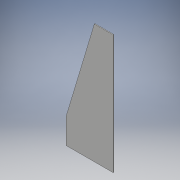
# Autodesk Inventor part: Part2
Saved by Autodesk Inventor 2018 (Build 220112000, 112)
## iProperties
Created: 2018-06-07
Part Number: Part2
Material: 一般
Document SubType Name: Modeling
Designer: ku_sk
Density: 1 g/cm^3
Appearance: 既定
Author: ku_sk
Autodesk Inventor part; units mm, degrees
ref_plane "YZ Plane" through (0, 0, 0) normal (1, 0, 0) x (0, 1, 0)
ref_plane "XZ Plane" through (0, 0, 0) normal (0, 1, 0) x (-1, 0, 0)
ref_plane "XY Plane" through (0, 0, 0) normal (0, 0, 1) x (1, 0, 0)
sketch "スケッチ1" plane through (0, 0, 0) normal (0, 1, 0) x (-1, 0, 0)
  line L0 (0, 254.5) -> (0, -254.5)
  line L1 (0, -254.5) -> (200, -254.5)
  line L2 (200, -254.5) -> (200, -145.5)
  line L3 (200, -145.5) -> (80, 254.5)
  line L4 (80, 254.5) -> (0, 254.5)
  point P0 (0, 0)
  point P1 (0, 0)
  dimension "d0" = 509
  dimension "d1" = 200
  dimension "d2" = 109
  dimension "d3" = 80
  constraints: 10 end point, 2 perpendicular, 1 coincident, 1 midpoint, 1 parallel, 1 vertical
  measures "d0" distance of L0.start L0.end
  measures "d1" distance of L0.end L1.end
  measures "d2" distance of L1.end L2.end
  measures "d3" distance of L3.end L0.start
extrude "押し出し1" add sketch "スケッチ1" along normal blind 3
